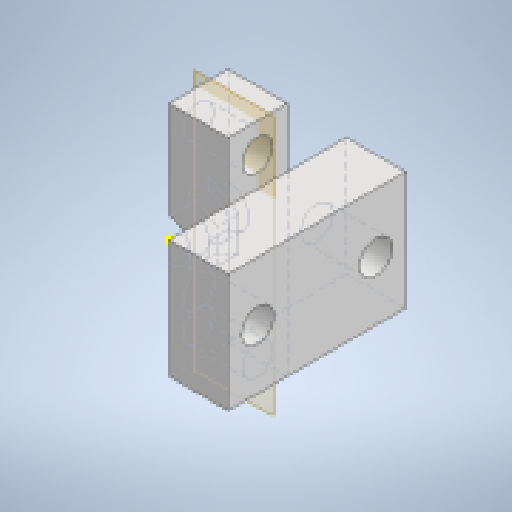
# Autodesk Inventor part: POMSliderMotor
Saved by Autodesk Inventor 2023 (Build 270158000, 158)
## iProperties
Created: 2023-03-27
Part Number: POMSliderMotor
Material: Generic
Document SubType Name: Modeling
Designer: Nathann
Density: 1 g/cm^3
Appearance: Default
Author: Nathann
Autodesk Inventor part; units mm, degrees
ref_plane "YZ Plane" through (0, 0, 0) normal (1, 0, 0) x (0, 1, 0)
ref_plane "XZ Plane" through (0, 0, 0) normal (0, 1, 0) x (-1, 0, 0)
ref_plane "XY Plane" through (0, 0, 0) normal (0, 0, 1) x (1, 0, 0)
sketch "Sketch1" plane through (0, 0, 0) normal (0, 0, 1) x (1, 0, 0)
  line L0 (10, -10) -> (-10, -10)
  line L1 (-10, -10) -> (-10, 10)
  line L2 (-10, 10) -> (10, 10)
  line L3 (10, 10) -> (10, -10)
  line L4 (10, -10) -> (-10, 10) construction
  line L5 (-10, -10) -> (10, 10) construction
  line L6 (10, -10) -> (6, -10)
  line L7 (6, 10) -> (10, 10)
  line L8 (10, 10) -> (10, -10)
  line L9 (0, 10) -> (0, -10)
  line L10 (0, -10) -> (0, 10)
  point P0 (0, 0)
  dimension "d0" = 20
  dimension "d1" = 20
  constraints: 22 end point, 4 midpoint, 3 parallel, 2 horizontal, 2 perpendicular, 2 point on line
  measures "d0" distance of L1.end L2.end
  measures "d1" distance of L0.end L1.end
extrude "Extrusion1" add sketch "Sketch1" along normal blind 5 contours L0 L9 L2 L3
ref_plane "Work Plane1" through (0, 0, 2.5) normal (0, 0, 1) x (1, 0, 0)
sketch "Sketch2" plane through (0, 0, 2.5) normal (0, 0, 1) x (1, 0, 0)
  line L0 (0, 10) -> (0, -10) projected
  line L1 (0, 2.8868) -> (2.5, 1.4434)
  line L2 (2.5, 1.4434) -> (2.5, -1.4434)
  line L3 (2.5, -1.4434) -> (0, -2.8868)
  line L4 (0, -2.8868) -> (-2.5, -1.4434)
  line L5 (-2.5, -1.4434) -> (-2.5, 1.4434)
  line L6 (-2.5, 1.4434) -> (0, 2.8868)
  point P0 (0, 0)
  point P1 (0, 0)
  dimension "d12" = 5
  constraints: 12 end point, 1 coincident, 1 point on line, 13 other
  measures "d12" distance between parallel lines of L2 L5
extrude "Extrusion2" cut sketch "Sketch2" along normal mid plane 1.8
sketch "Sketch3" plane through (0, 0, 5) normal (0, 0, 1) x (1, 0, 0)
  circle A0 centre (0, 0) radius 1.75
  dimension "d15" = 3.5
  constraints: 1 centre point, 1 coincident
  measures "d15" diameter of A0
extrude "Extrusion3" cut sketch "Sketch3" against normal blind 8
sketch "Sketch4" plane through (10, -10, 0) normal (1, 0, 0) x (0, 0, -1)
  circle A0 centre (-2.5, 17.5) radius 1.3
  circle A1 centre (-2.5, 2.5) radius 1.3
  line L0 (0, 20) -> (-5, 20) projected
  line L1 (0, 0) -> (-5, 0) projected
  line L2 (0, 0) -> (0, 20) projected
  point P0 (0, 10)
  dimension "d18" = 2.5
  dimension "d19" = 2.5
  dimension "d20" = 2.5
  dimension "d21" = 2.5
  dimension "d22" = 2.6
  dimension "d23" = 2.6
  constraints: 2 centre point
  measures "d18" distance from line of L0 A0.centre
  measures "d19" distance from line of L1 A1.centre
  measures "d20" distance from line of L2 A1.centre
  measures "d21" distance from line of L2 A0.centre
  measures "d22" diameter of A0
  measures "d23" diameter of A1
extrude "Extrusion4" cut sketch "Sketch4" against normal blind 25
sketch "Sketch5" plane through (10, -10, 0) normal (1, 0, 0) x (0, 0, -1)
  circle A0 centre (-2.5, 17.5) radius 1.3 projected
  circle A1 centre (-2.5, 17.5) radius 2
  circle A2 centre (-2.5, 2.5) radius 1.3 projected
  circle A3 centre (-2.5, 2.5) radius 2
  point P0 (0, 10)
  dimension "d26" = 4
  dimension "d27" = 4
  constraints: 2 centre point, 2 coincident
  measures "d26" diameter of A1
  measures "d27" diameter of A3
extrude "Extrusion5" cut sketch "Sketch5" against normal blind 4 contours A0 | A1 | A2 | A3
sketch "Sketch6" plane through (0, 0, 5) normal (0, 0, 1) x (1, 0, 0)
  point P0 (0, 0)
sketch "Sketch7" plane through (0, 0, 5) normal (0, 0, 1) x (1, 0, 0)
  line L0 (10, -10) -> (10, 10) projected
  line L1 (10, 10) -> (5, 10)
  line L2 (5, 10) -> (5, 5)
  line L3 (5, 5) -> (10, 5)
  line L4 (10, 5) -> (10, 10)
  line L5 (0, -10) -> (10, -10) projected
  line L6 (10, -10) -> (5, -10)
  line L7 (5, -10) -> (5, -5)
  line L8 (5, -5) -> (10, -5)
  line L9 (10, -5) -> (10, -10)
  point P0 (0, 0)
  dimension "d30" = 5
  dimension "d31" = 5
  dimension "d32" = 5
  dimension "d33" = 5
  constraints: 16 end point, 4 parallel, 2 horizontal, 2 perpendicular
  measures "d30" distance between parallel lines of L1 L3
  measures "d31" distance between parallel lines of L2 L0
  measures "d32" distance between parallel lines of L5 L8
  measures "d33" distance between parallel lines of L7 L0
extrude "Extrusion6" cut sketch "Sketch7" against normal blind 10
sketch "Sketch8" plane through (10, -5, 0) normal (1, 0, 0) x (0, 0, -1)
  line L0 (0, 0) -> (5, 0)
  line L1 (5, 0) -> (5, 10)
  line L2 (5, 10) -> (0, 10)
  line L3 (0, 10) -> (0, 0)
  line L4 (-5, 0) -> (-5, 10) projected
  line L5 (-5, 10) -> (-10, 10)
  line L6 (-10, 10) -> (-10, 0)
  line L7 (-10, 0) -> (-5, 0)
  line L8 (-5, 0) -> (-5, 10)
  circle A0 centre (-7.5, 5) radius 1.375
  circle A1 centre (2.5, 5) radius 1.375
  point P0 (0, 5)
  point P1 (-7.5, 0)
  dimension "d36" = 5
  dimension "d37" = 5
  dimension "d38" = 5
  dimension "d39" = 2.75
  dimension "d40" = 2.75
  dimension "d41" = 5
  dimension "d42" = 5
  dimension "d43" = 5
  dimension "d44" = 5
  dimension "d45" = 2.5
  dimension "d46" = 2.5
  constraints: 16 end point, 4 parallel, 2 centre point, 2 horizontal, 2 perpendicular, 1 midpoint, 1 point on line
  measures "d36" distance between parallel lines of L4 L6
  measures "d37" distance between parallel lines of L3 L4
  measures "d38" distance between parallel lines of L3 L1
  measures "d39" diameter of A0
  measures "d40" diameter of A1
  measures "d41" distance of point (-7.5, 0) A0.centre
  measures "d42" distance from line of L2 A1.centre
  measures "d43" distance from line of L0 A1.centre
  measures "d44" distance from line of L5 A0.centre
  measures "d45" distance from line of L4 A0.centre
  measures "d46" distance from line of L3 A1.centre
extrude "Extrusion7" add sketch "Sketch8" against normal blind 5
sketch "Sketch9" plane through (5, -5, 0) normal (-1, 0, 0) x (0, 0, 1)
  circle A0 centre (7.5, 5) radius 1.375 projected
  circle A1 centre (7.5, 5) radius 2
  circle A2 centre (-2.5, 5) radius 1.375 projected
  circle A3 centre (-2.5, 5) radius 2
  point P0 (0, 5)
  dimension "d49" = 4
  dimension "d50" = 4
  constraints: 2 centre point, 2 coincident
  measures "d49" diameter of A1
  measures "d50" diameter of A3
extrude "Extrusion8" cut sketch "Sketch9" against normal blind 2 contours A0 | A1 | A2 | A3
equation "\"d18\" = d19"
equation "\"d20\" = d19"
equation "\"d21\" = d19"
equation "\"d23\" = d22"
equation "\"d27\" = d26"
equation "\"d42\" = d41"
equation "\"d50\" = d49"
body "Solid1"
